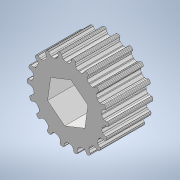
# Autodesk Inventor part: wheel_pulley
Saved by Autodesk Inventor 2022 (Build 260153000, 153)
## iProperties
Created: 2021-07-14
Part Number: wheel_pulley
Material: Generic
Document SubType Name: Modeling
Designer: gfellows
Density: 1 g/cm^3
Appearance: Default
Author: gfellows
Autodesk Inventor part; units mm, degrees
ref_plane "YZ Plane" through (0, 0, 0) normal (1, 0, 0) x (0, 1, 0)
ref_plane "XZ Plane" through (0, 0, 0) normal (0, 1, 0) x (-1, 0, 0)
ref_plane "XY Plane" through (0, 0, 0) normal (0, 0, 1) x (1, 0, 0)
sketch "Sketch1" plane through (0, 0, 0) normal (0, 0, 1) x (1, 0, 0)
  arc A0 (2.1993, -2.0799) -> (2.2142, -2.1983) centre (2.8796, -2.0546) ccw
  arc A1 (2.2558, -1.6304) -> (2.1993, -2.0799) centre (3.6004, -2.0277) ccw
  arc A2 (2.585, -0.955) -> (2.2558, -1.6304) centre (4.5816, -2.3459) ccw
  arc A3 (2.585, -0.955) -> (2.6265, -0.8778) centre (1.8842, -0.5284) ccw
  arc A4 (2.6265, -0.8778) -> (2.6045, -0.6145) centre (1.8188, -0.8127) ccw
  arc A5 (2.6045, -0.6145) -> (2.4177, -0.3797) centre (2.1396, -0.7927) ccw
  arc A6 (2.4177, -0.3797) -> (2.1605, -0.2382) centre (0.4564, -3.6402) ccw
  arc A7 (2.1605, -0.2382) -> (1.9007, -0.1016) centre (0.2608, -3.535) ccw
  arc A8 (1.9007, -0.1016) -> (1.6018, -0.0751) centre (1.7093, -0.5612) ccw
  arc A9 (1.6018, -0.0751) -> (1.37, -0.2018) centre (1.8694, -0.8399) ccw
  arc A10 (1.37, -0.2018) -> (1.3285, -0.2791) centre (2.0707, -0.6287) ccw
  arc A11 (0.9463, -0.9259) -> (1.3285, -0.2791) centre (-0.9325, 0.6205) ccw
  arc A12 (0.6023, -1.2208) -> (0.9463, -0.9259) centre (-0.1262, -0.0228) ccw
  arc A13 (0.4954, -1.2736) -> (0.6023, -1.2208) centre (0.2486, -0.6392) ccw
  arc A14 (-0.4954, -1.2736) -> (0.4954, -1.2736) centre (0, 0) ccw
  line L0 (-0.6754, -1.2114) -> (-0.4954, -1.2736)
  line L1 (-0.8571, -1.1541) -> (-0.6754, -1.2114)
  arc A15 (-1.6529, -0.564) -> (-0.8571, -1.1541) centre (-0.4964, 0.164) ccw
  arc A16 (-1.7074, -0.4578) -> (-1.6529, -0.564) centre (-1.0768, -0.2014) ccw
  arc A17 (-1.808, -0.0161) -> (-1.7074, -0.4578) centre (-0.4086, 0.0704) ccw
  arc A18 (-1.7297, 0.7311) -> (-1.808, -0.0161) centre (0.6222, 0.107) ccw
  arc A19 (-1.7297, 0.7311) -> (-1.7171, 0.8179) centre (-2.5341, 0.8924) ccw
  arc A20 (-1.7171, 0.8179) -> (-1.8278, 1.0578) centre (-2.4983, 0.6029) ccw
  arc A21 (-1.8278, 1.0578) -> (-2.0837, 1.2145) centre (-2.2037, 0.7314) ccw
  arc A22 (-2.0837, 1.2145) -> (-2.3737, 1.2595) centre (-2.8115, -2.5202) ccw
  arc A23 (-2.3737, 1.2595) -> (-2.6646, 1.299) centre (-3.0313, -2.4882) ccw
  arc A24 (-2.6646, 1.299) -> (-2.9545, 1.2217) centre (-2.6872, 0.8017) ccw
  arc A25 (-2.9545, 1.2217) -> (-3.129, 1.0234) centre (-2.4415, 0.5946) ccw
  arc A26 (-3.129, 1.0234) -> (-3.1416, 0.9366) centre (-2.3246, 0.8619) ccw
  arc A27 (-3.2795, 0.198) -> (-3.1416, 0.9366) centre (-5.5739, 1.0086) ccw
  arc A28 (-3.5019, -0.1967) -> (-3.2795, 0.198) centre (-4.5962, 0.6798) ccw
  arc A29 (-3.5844, -0.2829) -> (-3.5019, -0.1967) centre (-4.0332, 0.2289) ccw
  arc A30 (-4.5153, -0.6217) -> (-3.5844, -0.2829) centre (-4.4854, 0.7444) ccw
  line L2 (-4.7058, -0.6249) -> (-4.5153, -0.6217)
  line L3 (-4.8961, -0.6332) -> (-4.7058, -0.6249)
  arc A31 (-5.8458, -0.3508) -> (-4.8961, -0.6332) centre (-5.008, 0.7287) ccw
  arc A32 (-5.9332, -0.2697) -> (-5.8458, -0.3508) centre (-5.4284, 0.1869) ccw
  arc A33 (-6.1789, 0.111) -> (-5.9332, -0.2697) centre (-4.8935, 0.6709) ccw
  arc A34 (-6.3609, 0.8399) -> (-6.1789, 0.111) centre (-3.9373, 1.0578) ccw
  arc A35 (-6.3609, 0.8399) -> (-6.3787, 0.9257) centre (-7.1719, 0.7163) ccw
  arc A36 (-6.3787, 0.9257) -> (-6.5648, 1.1133) centre (-7.0393, 0.4565) ccw
  arc A37 (-6.5648, 1.1133) -> (-6.8588, 1.1731) centre (-6.8064, 0.678) ccw
  arc A38 (-6.8588, 1.1731) -> (-7.1468, 1.1161) centre (-6.2654, -2.5853) ccw
  arc A39 (-7.1468, 1.1161) -> (-7.4336, 1.0538) centre (-6.483, -2.6304) ccw
  arc A40 (-7.4336, 1.0538) -> (-7.6796, 0.882) centre (-7.2848, 0.5787) ccw
  arc A41 (-7.6796, 0.882) -> (-7.7757, 0.6359) centre (-6.983, 0.4681) ccw
  arc A42 (-7.7757, 0.6359) -> (-7.7579, 0.55) centre (-6.9646, 0.7593) ccw
  arc A43 (-7.6349, -0.1911) -> (-7.7579, 0.55) centre (-10.0681, -0.2141) ccw
  arc A44 (-7.7089, -0.6381) -> (-7.6349, -0.1911) centre (-9.037, -0.1888) ccw
  arc A45 (-7.7569, -0.7473) -> (-7.7089, -0.6381) centre (-8.3537, -0.4199) ccw
  arc A46 (-8.5158, -1.3841) -> (-7.7569, -0.7473) centre (-8.955, -0.0901) ccw
  line L4 (-8.6937, -1.4523) -> (-8.5158, -1.3841)
  line L5 (-8.8697, -1.5251) -> (-8.6937, -1.4523)
  arc A47 (-9.8587, -1.5846) -> (-8.8697, -1.5251) centre (-9.4406, -0.2836) ccw
  arc A48 (-9.9686, -1.5383) -> (-9.8587, -1.5846) centre (-9.6504, -0.9365) ccw
  arc A49 (-10.3296, -1.2646) -> (-9.9686, -1.5383) centre (-9.3133, -0.2988) ccw
  arc A50 (-10.75, -0.6419) -> (-10.3296, -1.2646) centre (-8.5471, 0.3918) ccw
  arc A51 (-10.75, -0.6419) -> (-10.7961, -0.5673) centre (-11.4698, -1.0354) ccw
  arc A52 (-10.7961, -0.5673) -> (-11.0351, -0.4547) centre (-11.2563, -1.2342) ccw
  arc A53 (-11.0351, -0.4547) -> (-11.3318, -0.4991) centre (-11.1132, -0.9464) ccw
  arc A54 (-11.3318, -0.4991) -> (-11.5829, -0.6511) centre (-9.4888, -3.8278) ccw
  arc A55 (-11.5829, -0.6511) -> (-11.8312, -0.8078) centre (-9.6778, -3.9447) ccw
  arc A56 (-11.8312, -0.8078) -> (-12.0036, -1.0533) centre (-11.5288, -1.2033) ccw
  arc A57 (-12.0036, -1.0533) -> (-12.0097, -1.3174) centre (-11.2074, -1.204) ccw
  arc A58 (-12.0097, -1.3174) -> (-11.9636, -1.392) centre (-11.2897, -0.9241) ccw
  arc A59 (-11.5945, -2.0464) -> (-11.9636, -1.392) centre (-13.8731, -2.9003) ccw
  arc A60 (-11.5112, -2.4918) -> (-11.5945, -2.0464) centre (-12.9129, -2.5238) ccw
  arc A61 (-11.5189, -2.6108) -> (-11.5112, -2.4918) centre (-12.1917, -2.5073) ccw
  arc A62 (-12.0142, -3.4688) -> (-11.5189, -2.6108) centre (-12.8695, -2.403) ccw
  line L6 (-12.1581, -3.5937) -> (-12.0142, -3.4688)
  line L7 (-12.2986, -3.7223) -> (-12.1581, -3.5937)
  arc A63 (-13.2076, -4.1165) -> (-12.2986, -3.7223) centre (-13.2597, -2.7509) ccw
  arc A64 (-13.3267, -4.1105) -> (-13.2076, -4.1165) centre (-13.2336, -3.4362) ccw
  arc A65 (-13.7596, -3.9768) -> (-13.3267, -4.1105) centre (-13.1348, -2.7217) ccw
  arc A66 (-14.3676, -3.5354) -> (-13.7596, -3.9768) centre (-12.6511, -1.8107) ccw
  arc A67 (-14.3676, -3.5354) -> (-14.4364, -3.4811) centre (-14.9094, -4.1514) ccw
  arc A68 (-14.4364, -3.4811) -> (-14.6995, -3.457) centre (-14.6408, -4.2652) ccw
  arc A69 (-14.6995, -3.457) -> (-14.9631, -3.6003) centre (-14.6047, -3.9458) ccw
  arc A70 (-14.9631, -3.6003) -> (-15.1471, -3.829) centre (-12.0927, -6.0979) ccw
  arc A71 (-15.1471, -3.829) -> (-15.3268, -4.0611) centre (-12.2304, -6.2723) ccw
  arc A72 (-15.3268, -4.0611) -> (-15.4048, -4.3508) centre (-14.9075, -4.3294) ccw
  arc A73 (-15.4048, -4.3508) -> (-15.3203, -4.6011) centre (-14.6052, -4.2201) ccw
  arc A74 (-15.3203, -4.6011) -> (-15.2514, -4.6554) centre (-14.7782, -3.9853) ccw
  arc A75 (-14.6808, -5.1441) -> (-15.2514, -4.6554) centre (-16.5299, -6.7258) ccw
  arc A76 (-14.4501, -5.5341) -> (-14.6808, -5.1441) centre (-15.7564, -6.0436) ccw
  arc A77 (-14.4167, -5.6486) -> (-14.4501, -5.5341) centre (-15.0843, -5.7814) ccw
  arc A78 (-14.5887, -6.6243) -> (-14.4167, -5.6486) centre (-15.7569, -5.9153) ccw
  line L8 (-14.6812, -6.7908) -> (-14.5887, -6.6243)
  line L9 (-14.7692, -6.9598) -> (-14.6812, -6.7908)
  arc A79 (-15.4886, -7.641) -> (-14.7692, -6.9598) centre (-16.0046, -6.3757) ccw
  arc A80 (-15.6026, -7.6762) -> (-15.4886, -7.641) centre (-15.7456, -7.0107) ccw
  arc A81 (-16.0551, -7.6986) -> (-15.6026, -7.6762) centre (-15.8973, -6.3055) ccw
  arc A82 (-16.7773, -7.4918) -> (-16.0551, -7.6986) centre (-15.7543, -5.284) ccw
  arc A83 (-16.7773, -7.4918) -> (-16.8606, -7.4643) centre (-17.0758, -8.256) ccw
  arc A84 (-16.8606, -7.4643) -> (-17.116, -7.5316) centre (-16.7845, -8.271) ccw
  arc A85 (-17.116, -7.5316) -> (-17.3148, -7.7564) centre (-16.8599, -7.9585) ccw
  arc A86 (-17.3148, -7.7564) -> (-17.4095, -8.0342) centre (-13.7633, -9.1217) ccw
  arc A87 (-17.4095, -8.0342) -> (-17.499, -8.3138) centre (-13.833, -9.3326) ccw
  arc A88 (-17.499, -8.3138) -> (-17.4732, -8.6128) centre (-17.0131, -8.4225) ccw
  arc A89 (-17.4732, -8.6128) -> (-17.3081, -8.819) centre (-16.7665, -8.2164) ccw
  arc A90 (-17.3081, -8.819) -> (-17.2248, -8.8465) centre (-17.0094, -8.0549) ccw
  arc A91 (-16.5215, -9.1106) -> (-17.2248, -8.8465) centre (-17.7181, -11.2293) ccw
  arc A92 (-16.1713, -9.3981) -> (-16.5215, -9.1106) centre (-17.2246, -10.3237) ccw
  arc A93 (-16.1007, -9.4943) -> (-16.1713, -9.3981) centre (-16.6827, -9.8475) ccw
  arc A94 (-15.9287, -10.47) -> (-16.1007, -9.4943) centre (-17.269, -10.2033) ccw
  line L10 (-15.9587, -10.6581) -> (-15.9287, -10.47)
  line L11 (-15.9836, -10.847) -> (-15.9587, -10.6581)
  arc A95 (-16.4265, -11.7332) -> (-15.9836, -10.847) centre (-17.3442, -10.7206) ccw
  arc A96 (-16.5216, -11.8052) -> (-16.4265, -11.7332) centre (-16.8837, -11.2288) ccw
  arc A97 (-16.9392, -11.981) -> (-16.5216, -11.8052) centre (-17.2674, -10.6179) ccw
  arc A98 (-17.6886, -12.0337) -> (-16.9392, -11.981) centre (-17.4824, -9.6091) ccw
  arc A99 (-17.6886, -12.0337) -> (-17.7763, -12.0363) centre (-17.7077, -12.8539) ccw
  arc A100 (-17.7763, -12.0363) -> (-17.9933, -12.187) centre (-17.4288, -12.7683) ccw
  arc A101 (-17.9933, -12.187) -> (-18.1032, -12.4662) centre (-17.6065, -12.5005) ccw
  arc A102 (-18.1032, -12.4662) -> (-18.0971, -12.7597) centre (-14.2989, -12.5344) ccw
  arc A103 (-18.0971, -12.7597) -> (-18.0856, -13.053) centre (-14.2922, -12.7565) ccw
  arc A104 (-18.0856, -13.053) -> (-17.9591, -13.3251) centre (-17.5919, -12.9889) ccw
  arc A105 (-17.9591, -13.3251) -> (-17.7334, -13.4624) centre (-17.4306, -12.7109) ccw
  arc A106 (-17.7334, -13.4624) -> (-17.6458, -13.4598) centre (-17.7141, -12.6423) ccw
  arc A107 (-16.8945, -13.4674) -> (-17.6458, -13.4598) centre (-17.2944, -15.8676) ccw
  arc A108 (-16.4672, -13.6178) -> (-16.8945, -13.4674) centre (-17.1403, -14.8478) ccw
  arc A109 (-16.3679, -13.6841) -> (-16.4672, -13.6178) centre (-16.794, -14.215) ccw
  arc A110 (-15.8726, -14.542) -> (-16.3679, -13.6841) centre (-17.2232, -14.7498) ccw
  line L12 (-15.8364, -14.7291) -> (-15.8726, -14.542)
  line L13 (-15.7952, -14.9151) -> (-15.8364, -14.7291)
  arc A111 (-15.9083, -15.8993) -> (-15.7952, -14.9151) centre (-17.117, -15.2617) ccw
  arc A112 (-15.973, -15.9996) -> (-15.9083, -15.8993) centre (-16.5104, -15.5817) ccw
  arc A113 (-16.3053, -16.3076) -> (-15.973, -15.9996) centre (-17.0799, -15.1389) ccw
  arc A114 (-16.9915, -16.6134) -> (-16.3053, -16.3076) centre (-17.627, -14.2645) ccw
  arc A115 (-16.9915, -16.6134) -> (-17.073, -16.6459) centre (-16.729, -17.3907) ccw
  arc A116 (-17.073, -16.6459) -> (-17.2254, -16.8617) centre (-16.4962, -17.2149) ccw
  arc A117 (-17.2254, -16.8617) -> (-17.2332, -17.1616) centre (-16.7547, -17.024) ccw
  arc A118 (-17.2332, -17.1616) -> (-17.1271, -17.4353) centre (-13.635, -15.9246) ccw
  arc A119 (-17.1271, -17.4353) -> (-17.0159, -17.707) centre (-13.5527, -16.131) ccw
  arc A120 (-17.0159, -17.707) -> (-16.804, -17.9194) centre (-16.5739, -17.4779) ccw
  arc A121 (-16.804, -17.9194) -> (-16.545, -17.9713) centre (-16.5174, -17.1615) ccw
  arc A122 (-16.545, -17.9713) -> (-16.4635, -17.9389) centre (-16.8073, -17.194) ccw
  arc A123 (-15.755, -17.689) -> (-16.4635, -17.9389) centre (-15.3098, -20.0813) ccw
  arc A124 (-15.3019, -17.6842) -> (-15.755, -17.689) centre (-15.5138, -19.0702) ccw
  arc A125 (-15.186, -17.7125) -> (-15.3019, -17.6842) centre (-15.4048, -18.3571) ccw
  arc A126 (-14.4271, -18.3494) -> (-15.186, -17.7125) centre (-15.6252, -19.0066) ccw
  line L14 (-14.3291, -18.5127) -> (-14.4271, -18.3494)
  line L15 (-14.2268, -18.6734) -> (-14.3291, -18.5127)
  arc A127 (-13.9965, -19.637) -> (-14.2268, -18.6734) centre (-15.3503, -19.4513) ccw
  arc A128 (-14.023, -19.7533) -> (-13.9965, -19.637) centre (-14.6709, -19.5445) ccw
  arc A129 (-14.2298, -20.1564) -> (-14.023, -19.7533) centre (-15.3575, -19.3232) ccw
  arc A130 (-14.7701, -20.6785) -> (-14.2298, -20.1564) centre (-16.1706, -18.6886) ccw
  arc A131 (-14.7701, -20.6785) -> (-14.8356, -20.7368) centre (-14.2576, -21.3191) ccw
  arc A132 (-14.8356, -20.7368) -> (-14.905, -20.9917) centre (-14.0989, -21.0743) ccw
  arc A133 (-14.905, -20.9917) -> (-14.8097, -21.2763) centre (-14.4072, -20.9833) ccw
  arc A134 (-14.8097, -21.2763) -> (-14.6164, -21.4972) centre (-11.8516, -18.8832) ccw
  arc A135 (-14.6164, -21.4972) -> (-14.419, -21.7145) centre (-11.7037, -19.049) ccw
  arc A136 (-14.419, -21.7145) -> (-14.1472, -21.8416) centre (-14.082, -21.348) ccw
  arc A137 (-14.1472, -21.8416) -> (-13.8861, -21.8018) centre (-14.1371, -21.0314) ccw
  arc A138 (-13.8861, -21.8018) -> (-13.8206, -21.7434) centre (-14.3984, -21.161) ccw
  arc A139 (-13.2402, -21.2663) -> (-13.8206, -21.7434) centre (-12.0037, -23.362) ccw
  arc A140 (-12.8162, -21.1069) -> (-13.2402, -21.2663) centre (-12.5413, -22.4817) ccw
  arc A141 (-12.6976, -21.0938) -> (-12.8162, -21.1069) centre (-12.6827, -21.7744) ccw
  arc A142 (-11.7666, -21.4327) -> (-12.6976, -21.0938) centre (-12.6677, -22.46) ccw
  line L16 (-11.6187, -21.5527) -> (-11.7666, -21.4327)
  line L17 (-11.4675, -21.6687) -> (-11.6187, -21.5527)
  arc A143 (-10.9216, -22.4954) -> (-11.4675, -21.6687) centre (-12.2573, -22.7839) ccw
  arc A144 (-10.9067, -22.6138) -> (-10.9216, -22.4954) centre (-11.5869, -22.6391) ccw
  arc A145 (-10.9632, -23.0633) -> (-10.9067, -22.6138) centre (-12.3078, -22.666) ccw
  arc A146 (-11.2923, -23.7386) -> (-10.9632, -23.0633) centre (-13.2889, -22.3477) ccw
  arc A147 (-11.2923, -23.7386) -> (-11.3339, -23.8159) centre (-10.5916, -24.1653) ccw
  arc A148 (-11.3339, -23.8159) -> (-11.3119, -24.0791) centre (-10.5262, -23.881) ccw
  arc A149 (-11.3119, -24.0791) -> (-11.1251, -24.3139) centre (-10.847, -23.901) ccw
  arc A150 (-11.1251, -24.3139) -> (-10.8679, -24.4554) centre (-9.1638, -21.0534) ccw
  arc A151 (-10.8679, -24.4554) -> (-10.6081, -24.5921) centre (-8.9682, -21.1587) ccw
  arc A152 (-10.6081, -24.5921) -> (-10.3092, -24.6186) centre (-10.4167, -24.1325) ccw
  arc A153 (-10.3092, -24.6186) -> (-10.0774, -24.4918) centre (-10.5768, -23.8538) ccw
  arc A154 (-10.0774, -24.4918) -> (-10.0359, -24.4146) centre (-10.778, -24.065) ccw
  arc A155 (-9.6537, -23.7678) -> (-10.0359, -24.4146) centre (-7.7749, -25.3142) ccw
  arc A156 (-9.3097, -23.4729) -> (-9.6537, -23.7678) centre (-8.5811, -24.6708) ccw
  arc A157 (-9.2027, -23.4201) -> (-9.3097, -23.4729) centre (-8.956, -24.0545) ccw
  arc A158 (-8.212, -23.4201) -> (-9.2027, -23.4201) centre (-8.7074, -24.6937) ccw
  line L18 (-8.0319, -23.4823) -> (-8.212, -23.4201)
  line L19 (-7.8503, -23.5396) -> (-8.0319, -23.4823)
  arc A159 (-7.0545, -24.1297) -> (-7.8503, -23.5396) centre (-8.211, -24.8576) ccw
  arc A160 (-7, -24.2358) -> (-7.0545, -24.1297) centre (-7.6306, -24.4923) ccw
  arc A161 (-6.8994, -24.6776) -> (-7, -24.2358) centre (-8.2988, -24.7641) ccw
  arc A162 (-6.9777, -25.4248) -> (-6.8994, -24.6776) centre (-9.3296, -24.8007) ccw
  arc A163 (-6.9777, -25.4248) -> (-6.9903, -25.5116) centre (-6.1733, -25.586) ccw
  arc A164 (-6.9903, -25.5116) -> (-6.8796, -25.7514) centre (-6.2091, -25.2965) ccw
  arc A165 (-6.8796, -25.7514) -> (-6.6237, -25.9082) centre (-6.5037, -25.425) ccw
  arc A166 (-6.6237, -25.9082) -> (-6.3336, -25.9532) centre (-5.8959, -22.1735) ccw
  arc A167 (-6.3336, -25.9532) -> (-6.0428, -25.9927) centre (-5.676, -22.2055) ccw
  arc A168 (-6.0428, -25.9927) -> (-5.7529, -25.9154) centre (-6.0201, -25.4954) ccw
  arc A169 (-5.7529, -25.9154) -> (-5.5784, -25.717) centre (-6.2659, -25.2883) ccw
  arc A170 (-5.5784, -25.717) -> (-5.5658, -25.6303) centre (-6.3828, -25.5556) ccw
  arc A171 (-5.4279, -24.8917) -> (-5.5658, -25.6303) centre (-3.1335, -25.7023) ccw
  arc A172 (-5.2055, -24.497) -> (-5.4279, -24.8917) centre (-4.1111, -25.3735) ccw
  arc A173 (-5.123, -24.4108) -> (-5.2055, -24.497) centre (-4.6742, -24.9225) ccw
  arc A174 (-4.1921, -24.0719) -> (-5.123, -24.4108) centre (-4.222, -25.4381) ccw
  line L20 (-4.0016, -24.0687) -> (-4.1921, -24.0719)
  line L21 (-3.8112, -24.0605) -> (-4.0016, -24.0687)
  arc A175 (-2.8616, -24.3428) -> (-3.8112, -24.0605) centre (-3.6994, -25.4224) ccw
  arc A176 (-2.7741, -24.424) -> (-2.8616, -24.3428) centre (-3.2789, -24.8806) ccw
  arc A177 (-2.5285, -24.8046) -> (-2.7741, -24.424) centre (-3.8139, -25.3646) ccw
  arc A178 (-2.3465, -25.5335) -> (-2.5285, -24.8046) centre (-4.77, -25.7514) ccw
  arc A179 (-2.3465, -25.5335) -> (-2.3287, -25.6194) centre (-1.5354, -25.4099) ccw
  arc A180 (-2.3287, -25.6194) -> (-2.1426, -25.8069) centre (-1.6681, -25.1502) ccw
  arc A181 (-2.1426, -25.8069) -> (-1.8486, -25.8667) centre (-1.901, -25.3717) ccw
  arc A182 (-1.8486, -25.8667) -> (-1.5606, -25.8098) centre (-2.442, -22.1084) ccw
  arc A183 (-1.5606, -25.8098) -> (-1.2737, -25.7475) centre (-2.2244, -22.0632) ccw
  arc A184 (-1.2737, -25.7475) -> (-1.0278, -25.5757) centre (-1.4226, -25.2724) ccw
  arc A185 (-1.0278, -25.5757) -> (-0.9317, -25.3296) centre (-1.7244, -25.1618) ccw
  arc A186 (-0.9317, -25.3296) -> (-0.9495, -25.2437) centre (-1.7427, -25.453) ccw
  arc A187 (-1.0725, -24.5026) -> (-0.9495, -25.2437) centre (1.3607, -24.4795) ccw
  arc A188 (-0.9985, -24.0556) -> (-1.0725, -24.5026) centre (0.3296, -24.5049) ccw
  arc A189 (-0.9505, -23.9463) -> (-0.9985, -24.0556) centre (-0.3537, -24.2737) ccw
  arc A190 (-0.1916, -23.3095) -> (-0.9505, -23.9463) centre (0.2476, -24.6036) ccw
  line L22 (-0.0137, -23.2414) -> (-0.1916, -23.3095)
  line L23 (0.1623, -23.1685) -> (-0.0137, -23.2414)
  arc A191 (1.1513, -23.1091) -> (0.1623, -23.1685) centre (0.7333, -24.4101) ccw
  arc A192 (1.2612, -23.1554) -> (1.1513, -23.1091) centre (0.943, -23.7572) ccw
  arc A193 (1.6223, -23.4291) -> (1.2612, -23.1554) centre (0.6059, -24.3949) ccw
  arc A194 (2.0426, -24.0518) -> (1.6223, -23.4291) centre (-0.1603, -25.0854) ccw
  arc A195 (2.0426, -24.0518) -> (2.0887, -24.1264) centre (2.7624, -23.6583) ccw
  arc A196 (2.0887, -24.1264) -> (2.3277, -24.239) centre (2.5489, -23.4595) ccw
  arc A197 (2.3277, -24.239) -> (2.6244, -24.1946) centre (2.4058, -23.7473) ccw
  arc A198 (2.6244, -24.1946) -> (2.8756, -24.0426) centre (0.7814, -20.8658) ccw
  arc A199 (2.8756, -24.0426) -> (3.1238, -23.8859) centre (0.9704, -20.749) ccw
  arc A200 (3.1238, -23.8859) -> (3.2962, -23.6403) centre (2.8215, -23.4904) ccw
  arc A201 (3.2962, -23.6403) -> (3.3023, -23.3762) centre (2.5, -23.4897) ccw
  arc A202 (3.3023, -23.3762) -> (3.2562, -23.3016) centre (2.5824, -23.7696) ccw
  arc A203 (2.8871, -22.6472) -> (3.2562, -23.3016) centre (5.1657, -21.7934) ccw
  arc A204 (2.8038, -22.2019) -> (2.8871, -22.6472) centre (4.2055, -22.1699) ccw
  arc A205 (2.8115, -22.0829) -> (2.8038, -22.2019) centre (3.4843, -22.1864) ccw
  arc A206 (3.3069, -21.2249) -> (2.8115, -22.0829) centre (4.1621, -22.2907) ccw
  line L24 (3.4507, -21.1) -> (3.3069, -21.2249)
  line L25 (3.5912, -20.9713) -> (3.4507, -21.1)
  arc A207 (4.5002, -20.5772) -> (3.5912, -20.9713) centre (4.5523, -21.9427) ccw
  arc A208 (4.6193, -20.5831) -> (4.5002, -20.5772) centre (4.5262, -21.2574) ccw
  arc A209 (5.0522, -20.7168) -> (4.6193, -20.5831) centre (4.4274, -21.972) ccw
  arc A210 (5.6602, -21.1582) -> (5.0522, -20.7168) centre (3.9437, -22.883) ccw
  arc A211 (5.6602, -21.1582) -> (5.729, -21.2126) centre (6.202, -20.5422) ccw
  arc A212 (5.729, -21.2126) -> (5.9921, -21.2366) centre (5.9334, -20.4285) ccw
  arc A213 (5.9921, -21.2366) -> (6.2558, -21.0934) centre (5.8974, -20.7479) ccw
  arc A214 (6.2558, -21.0934) -> (6.4398, -20.8647) centre (3.3854, -18.5958) ccw
  arc A215 (6.4398, -20.8647) -> (6.6194, -20.6326) centre (3.523, -18.4214) ccw
  arc A216 (6.6194, -20.6326) -> (6.6974, -20.3428) centre (6.2001, -20.3643) ccw
  arc A217 (6.6974, -20.3428) -> (6.6129, -20.0926) centre (5.8978, -20.4736) ccw
  arc A218 (6.6129, -20.0926) -> (6.544, -20.0382) centre (6.0709, -20.7084) ccw
  arc A219 (5.9734, -19.5495) -> (6.544, -20.0382) centre (7.8226, -17.9678) ccw
  arc A220 (5.7428, -19.1596) -> (5.9734, -19.5495) centre (7.049, -18.6501) ccw
  arc A221 (5.7093, -19.0451) -> (5.7428, -19.1596) centre (6.3769, -18.9122) ccw
  arc A222 (5.8813, -18.0694) -> (5.7093, -19.0451) centre (7.0496, -18.7784) ccw
  line L26 (5.9738, -17.9028) -> (5.8813, -18.0694)
  line L27 (6.0618, -17.7339) -> (5.9738, -17.9028)
  arc A223 (6.7812, -17.0527) -> (6.0618, -17.7339) centre (7.2972, -18.318) ccw
  arc A224 (6.8952, -17.0175) -> (6.7812, -17.0527) centre (7.0383, -17.683) ccw
  arc A225 (7.3477, -16.995) -> (6.8952, -17.0175) centre (7.1899, -18.3882) ccw
  arc A226 (8.0699, -17.2019) -> (7.3477, -16.995) centre (7.0469, -19.4097) ccw
  arc A227 (8.0699, -17.2019) -> (8.1532, -17.2294) centre (8.3684, -16.4377) ccw
  arc A228 (8.1532, -17.2294) -> (8.4086, -17.162) centre (8.0771, -16.4227) ccw
  arc A229 (8.4086, -17.162) -> (8.6074, -16.9373) centre (8.1525, -16.7352) ccw
  arc A230 (8.6074, -16.9373) -> (8.7021, -16.6594) centre (5.0559, -15.572) ccw
  arc A231 (8.7021, -16.6594) -> (8.7916, -16.3798) centre (5.1256, -15.361) ccw
  arc A232 (8.7916, -16.3798) -> (8.7658, -16.0809) centre (8.3057, -16.2712) ccw
  arc A233 (8.7658, -16.0809) -> (8.6007, -15.8746) centre (8.0591, -16.4773) ccw
  arc A234 (8.6007, -15.8746) -> (8.5174, -15.8471) centre (8.302, -16.6387) ccw
  arc A235 (7.8141, -15.5831) -> (8.5174, -15.8471) centre (9.0107, -13.4643) ccw
  arc A236 (7.464, -15.2955) -> (7.8141, -15.5831) centre (8.5172, -14.37) ccw
  arc A237 (7.3934, -15.1994) -> (7.464, -15.2955) centre (7.9753, -14.8462) ccw
  arc A238 (7.2213, -14.2237) -> (7.3934, -15.1994) centre (8.5616, -14.4904) ccw
  line L28 (7.2513, -14.0356) -> (7.2213, -14.2237)
  line L29 (7.2762, -13.8467) -> (7.2513, -14.0356)
  arc A239 (7.7192, -12.9605) -> (7.2762, -13.8467) centre (8.6369, -13.973) ccw
  arc A240 (7.8142, -12.8885) -> (7.7192, -12.9605) centre (8.1763, -13.4649) ccw
  arc A241 (8.2318, -12.7126) -> (7.8142, -12.8885) centre (8.56, -14.0757) ccw
  arc A242 (8.9812, -12.66) -> (8.2318, -12.7126) centre (8.775, -15.0845) ccw
  arc A243 (8.9812, -12.66) -> (9.0689, -12.6573) centre (9.0003, -11.8398) ccw
  arc A244 (9.0689, -12.6573) -> (9.2859, -12.5067) centre (8.7215, -11.9253) ccw
  arc A245 (9.2859, -12.5067) -> (9.3958, -12.2275) centre (8.8992, -12.1932) ccw
  arc A246 (9.3958, -12.2275) -> (9.3897, -11.934) centre (5.5915, -12.1592) ccw
  arc A247 (9.3897, -11.934) -> (9.3782, -11.6407) centre (5.5848, -11.9372) ccw
  arc A248 (9.3782, -11.6407) -> (9.2517, -11.3686) centre (8.8845, -11.7047) ccw
  arc A249 (9.2517, -11.3686) -> (9.026, -11.2312) centre (8.7232, -11.9828) ccw
  arc A250 (9.026, -11.2312) -> (8.9384, -11.2338) centre (9.0067, -12.0514) ccw
  arc A251 (8.1871, -11.2263) -> (8.9384, -11.2338) centre (8.587, -8.826) ccw
  arc A252 (7.7598, -11.0758) -> (8.1871, -11.2263) centre (8.4329, -9.8459) ccw
  arc A253 (7.6606, -11.0096) -> (7.7598, -11.0758) centre (8.0866, -10.4787) ccw
  arc A254 (7.1652, -10.1516) -> (7.6606, -11.0096) centre (8.5158, -9.9438) ccw
  line L30 (7.129, -9.9646) -> (7.1652, -10.1516)
  line L31 (7.0878, -9.7786) -> (7.129, -9.9646)
  arc A255 (7.201, -8.7943) -> (7.0878, -9.7786) centre (8.4096, -9.4319) ccw
  arc A256 (7.2657, -8.6941) -> (7.201, -8.7943) centre (7.803, -9.112) ccw
  arc A257 (7.5979, -8.3861) -> (7.2657, -8.6941) centre (8.3725, -9.5547) ccw
  arc A258 (8.2841, -8.0803) -> (7.5979, -8.3861) centre (8.9196, -10.4292) ccw
  arc A259 (8.2841, -8.0803) -> (8.3656, -8.0478) centre (8.0216, -7.303) ccw
  arc A260 (8.3656, -8.0478) -> (8.518, -7.832) centre (7.7888, -7.4788) ccw
  arc A261 (8.518, -7.832) -> (8.5258, -7.5321) centre (8.0474, -7.6697) ccw
  arc A262 (8.5258, -7.5321) -> (8.4197, -7.2584) centre (4.9276, -8.7691) ccw
  arc A263 (8.4197, -7.2584) -> (8.3085, -6.9867) centre (4.8453, -8.5627) ccw
  arc A264 (8.3085, -6.9867) -> (8.0966, -6.7743) centre (7.8665, -7.2157) ccw
  arc A265 (8.0966, -6.7743) -> (7.8376, -6.7224) centre (7.81, -7.5322) ccw
  arc A266 (7.8376, -6.7224) -> (7.7561, -6.7548) centre (8.0999, -7.4997) ccw
  arc A267 (7.0476, -7.0046) -> (7.7561, -6.7548) centre (6.6024, -4.6124) ccw
  arc A268 (6.5945, -7.0094) -> (7.0476, -7.0046) centre (6.8064, -5.6235) ccw
  arc A269 (6.4786, -6.9811) -> (6.5945, -7.0094) centre (6.6974, -6.3365) ccw
  arc A270 (5.7197, -6.3443) -> (6.4786, -6.9811) centre (6.9178, -5.6871) ccw
  line L32 (5.6217, -6.1809) -> (5.7197, -6.3443)
  line L33 (5.5194, -6.0202) -> (5.6217, -6.1809)
  arc A271 (5.2891, -5.0567) -> (5.5194, -6.0202) centre (6.6429, -5.2424) ccw
  arc A272 (5.3156, -4.9403) -> (5.2891, -5.0567) centre (5.9635, -5.1492) ccw
  arc A273 (5.5225, -4.5373) -> (5.3156, -4.9403) centre (6.6501, -5.3705) ccw
  arc A274 (6.0627, -4.0152) -> (5.5225, -4.5373) centre (7.4632, -6.0051) ccw
  arc A275 (6.0627, -4.0152) -> (6.1282, -3.9568) centre (5.5502, -3.3746) ccw
  arc A276 (6.1282, -3.9568) -> (6.1976, -3.7019) centre (5.3915, -3.6194) ccw
  arc A277 (6.1976, -3.7019) -> (6.1023, -3.4174) centre (5.6998, -3.7103) ccw
  arc A278 (6.1023, -3.4174) -> (5.909, -3.1965) centre (3.1442, -5.8105) ccw
  arc A279 (5.909, -3.1965) -> (5.7116, -2.9792) centre (2.9963, -5.6446) ccw
  arc A280 (5.7116, -2.9792) -> (5.4398, -2.8521) centre (5.3746, -3.3456) ccw
  arc A281 (5.4398, -2.8521) -> (5.1787, -2.8919) centre (5.4297, -3.6623) ccw
  arc A282 (5.1787, -2.8919) -> (5.1132, -2.9503) centre (5.6911, -3.5326) ccw
  arc A283 (4.5329, -3.4274) -> (5.1132, -2.9503) centre (3.2963, -1.3316) ccw
  arc A284 (4.1088, -3.5868) -> (4.5329, -3.4274) centre (3.8339, -2.2119) ccw
  arc A285 (3.9902, -3.5999) -> (4.1088, -3.5868) centre (3.9753, -2.9193) ccw
  arc A286 (3.0592, -3.261) -> (3.9902, -3.5999) centre (3.9603, -2.2337) ccw
  line L34 (2.9113, -3.141) -> (3.0592, -3.261)
  line L35 (2.7602, -3.025) -> (2.9113, -3.141)
  arc A287 (2.2142, -2.1983) -> (2.7602, -3.025) centre (3.5499, -1.9098) ccw
  line L36 (-3.2936, -5.0619) -> (-10.1326, -7.7863)
  line L37 (2.4853, -9.6224) -> (-3.2936, -5.0619)
  line L38 (1.4252, -16.9074) -> (2.4853, -9.6224)
  line L39 (-5.4138, -19.6318) -> (1.4252, -16.9074)
  line L40 (-11.1927, -15.0713) -> (-5.4138, -19.6318)
  line L41 (-10.1326, -7.7863) -> (-11.1927, -15.0713)
  point P0 (0, 0)
  point P1 (-4.3537, -12.3468)
  constraints: 576 point on circle, 288 centre point, 84 end point
extrude "Extrusion1" add sketch "Sketch1" along normal blind 15.04
body "Solid1"
